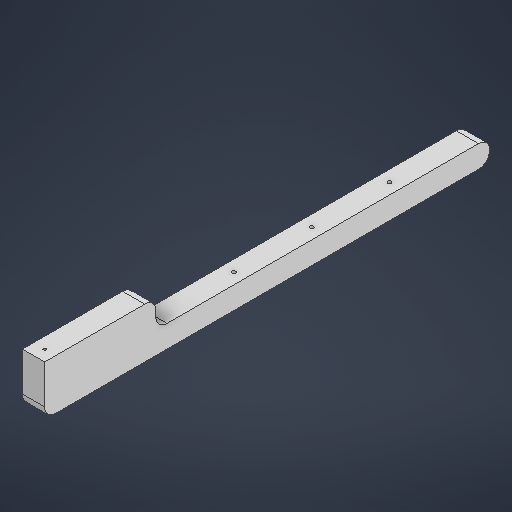
# Autodesk Inventor part: Aufhängung_Seitenteil_Koppeltest_außen
Saved by Autodesk Inventor 2027 (Build 310192060, 192F)
## iProperties
Created: 2026-07-21
Part Number: Aufhängung_Seitenteil_Koppeltest_außen
Material: Generic
Document SubType Name: Modeling
Designer: kw
Density: 1 g/cm^3
Appearance: Default
Author: kw
Autodesk Inventor part; units mm, degrees
ref_plane "YZ Plane" through (0, 0, 0) normal (1, 0, 0) x (0, 1, 0)
ref_plane "XZ Plane" through (0, 0, 0) normal (0, 1, 0) x (-1, 0, 0)
ref_plane "XY Plane" through (0, 0, 0) normal (0, 0, 1) x (1, 0, 0)
sketch "Sketch1" plane through (0, 0, 0) normal (0, 1, 0) x (-1, 0, 0)
  line L0 (0, 0) -> (20, 0)
  line L1 (20, 0) -> (20, -300)
  line L2 (20, -300) -> (0, -300)
  line L3 (0, -300) -> (0, 0)
  line L4 (0, -20) -> (0, 0)
  line L5 (0, 20) -> (0, 0)
  line L6 (0, 20) -> (45, 20)
  line L7 (45, 20) -> (45, 0)
  line L8 (45, 0) -> (20, 0)
  line L9 (20, -300) -> (45, -300)
  line L10 (45, -300) -> (45, -280)
  line L11 (45, -280) -> (20, -280)
  line L12 (0, 20) -> (45, 20)
  line L13 (45, 20) -> (45, 100)
  line L14 (45, 100) -> (0, 100)
  line L15 (0, 100) -> (0, 20)
  dimension "d32" = 20
  dimension "d33" = 300
  dimension "d100" = 45
  dimension "d101" = 25
  dimension "d102" = 20
  dimension "d103" = 80
  constraints: 32 end point, 5 parallel, 4 perpendicular, 3 horizontal, 1 point on line
  measures "d32" distance of L1.end L2.end
  measures "d33" distance of L0.end L1.end
  measures "d100" distance of L5.start L6.end
  measures "d101" distance of L1.end L9.end
  measures "d102" distance of L9.end L10.end
  measures "d103" distance of L13.end L12.end
extrude "Extrusion1" add sketch "Sketch1" along normal blind 20 contours L5 L6 L7 L8 L0 | L0 L1 L2 L3 | L15 L14 L13 L6
fillet "Fillet1" radius 10 5 edges at (0, 10, -300) (-45, 10, 0) (-20, 10, 0) (0, 10, 100) (-20, 10, -300)
sketch "Sketch10" plane through (0, 0, 100) normal (1, 0, 0) x (0, 0, -1)
  line L0 (390, 20) -> (390, 0) projected
  line L1 (390, 10) -> (320, 10)
  line L2 (320, 10) -> (250, 10)
  line L3 (250, 10) -> (180, 10)
  point P0 (100, 0)
  dimension "d104" = 70
  dimension "d105" = 70
  dimension "d106" = 70
  constraints: 6 end point, 2 point on line, 1 horizontal, 1 midpoint
  measures "d104" distance of L1.start L1.end
  measures "d105" distance of L1.end L2.end
  measures "d106" distance of L2.end L3.end
hole "Hole7" at (0, 10, -220) at (0, 10, -150) at (0, 10, -80) direction (-1, 0, 0) diameter 3.2 depth 20 clearance for "Socket Head Cap Screw ISO 4762" size "M3" standard "ISO"
sketch "Sketch11" plane through (-45, 0, 10) normal (-1, 0, 0) x (0, 0, 1)
  line L0 (90, 0) -> (90, 20) projected
  line L1 (90, 10) -> (80, 10)
  point P0 (-10, 0)
  dimension "d114" = 10
  constraints: 2 end point, 1 horizontal, 1 midpoint
  measures "d114" distance of L1.start L1.end
hole "Hole8" at (-45, 10, 90) direction (1, 0, 0) diameter 2.459 depth 8.8 tip angle 118 thread size "M3x0.5" class "6H" standard "ISO Metric profile"
body "Solid1"
